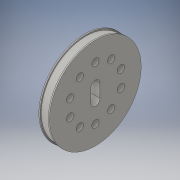
# Autodesk Inventor part: msheehan_wheel_small
Saved by Autodesk Inventor 2016 (Build 200138000, 138)
## iProperties
Created: 2017-09-05
Part Number: msheehan_wheel_small
Material: Generic
Document SubType Name: Modeling
Designer: Student
Density: 1 g/cm^3
Appearance: Default
Author: Student
Autodesk Inventor part; units mm, degrees
sketch "Sketch1" plane through (0, 0, 0) normal (1, 0, 0) x (0, 1, 0)
  circle A0 centre (0, 0) radius 23.368
  dimension "d0" = 46.736
  constraints: 1 centre point, 1 coincident
  measures "d0" diameter of A0
extrude "Extrusion1" add sketch "Sketch1" along normal blind 5.588
ref_plane "Work Plane2" through (5.588, 0, 0) normal (1, 0, 0) x (0, 0, -1)
sketch "Sketch3" plane through (5.588, 0, 0) normal (1, 0, 0) x (0, 0, -1)
  line L0 (0, -3.4925) -> (0, 3.4925) construction
  line L1 (2.413, -3.4925) -> (2.413, 3.4925)
  line L2 (-2.413, 3.4925) -> (-2.413, -3.4925)
  arc A0 (-2.413, -3.4925) -> (2.413, -3.4925) centre (0, -3.4925) ccw
  arc A1 (2.413, 3.4925) -> (-2.413, 3.4925) centre (0, 3.4925) ccw
  point P0 (0, 0)
  dimension "d8" = 3.4925
  dimension "d9" = 4.826
  constraints: 8 end point, 4 point on circle, 4 tangent, 2 centre point, 1 midpoint, 1 parallel, 1 vertical
  measures "d8" distance of point (0, 0) L0.end
  measures "d9" diameter of A1
extrude "Extrusion2" cut sketch "Sketch3" against normal blind 5.08
ref_plane "Work Plane3" through (5.588, 0, 0) normal (1, 0, 0) x (0, 0, -1)
sketch "Sketch6" plane through (5.588, 0, 0) normal (1, 0, 0) x (0, 0, -1)
  line L0 (0, 0) -> (0, 13.97)
  circle A0 centre (0, 13.97) radius 1.905
  circle A1 centre (-8.2114, 11.302) radius 1.905
  circle A2 centre (-13.2863, 4.317) radius 1.905
  circle A3 centre (-13.2863, -4.317) radius 1.905
  circle A4 centre (-8.2114, -11.302) radius 1.905
  circle A5 centre (0, -13.97) radius 1.905
  circle A6 centre (8.2114, -11.302) radius 1.905
  circle A7 centre (13.2863, -4.317) radius 1.905
  circle A8 centre (13.2863, 4.317) radius 1.905
  circle A9 centre (8.2114, 11.302) radius 1.905
  dimension "d16" = 13.97
  dimension "d17" = 3.81
  dimension "d20" = 360
  constraints: 10 centre point, 2 coincident, 2 end point, 1 vertical, 21 other
  measures "d16" distance of L0.start L0.end
  measures "d17" diameter of A0
extrude "Extrusion3" cut sketch "Sketch6" against normal blind 25.4
ref_plane "Work Plane1" through (5.588, 0, 0) normal (1, 0, 0) x (0, 0, -1)
sketch "Sketch7" plane through (5.588, 0, 0) normal (1, 0, 0) x (0, 0, -1)
  line L0 (0, 0) -> (0, -23.749) construction
  circle A0 centre (0, 0) radius 23.749 projected
  dimension "d24" = 23.749
  constraints: 2 end point, 1 vertical, 1 vertical alignment, 1 other
  measures "d24" distance of L0.start L0.end
sketch "Sketch8" plane through (0, 0, 0) normal (0, 1, 0) x (-1, 0, 0)
  line L0 (0, -23.368) -> (0, 23.368) projected
  line L1 (0, -23.368) -> (0, -24.003)
  line L2 (0, -24.003) -> (-0.635, -24.003)
  line L3 (-0.635, -24.003) -> (-0.635, -23.368)
  line L4 (-0.635, -23.368) -> (0, -23.368)
  line L5 (0, -23.368) -> (-5.588, -23.368) projected
  line L6 (-0.635, -23.368) -> (0, -23.368)
  line L7 (-5.588, -23.368) -> (-5.588, -24.003)
  line L8 (-5.588, -24.003) -> (-4.953, -24.003)
  line L9 (-4.953, -24.003) -> (-4.953, -23.368)
  line L10 (-4.953, -23.368) -> (-5.588, -23.368)
  line L11 (0, 0) -> (-5.8379, 0)
  dimension "d25" = 0.635
  dimension "d26" = 0.635
  dimension "d27" = 0.635
  dimension "d28" = 0.635
  constraints: 20 end point, 5 perpendicular, 2 collinear, 2 vertical, 1 horizontal, 1 point on line
  measures "d25" distance of L0.start L1.end
  measures "d26" distance of L1.end L2.end
  measures "d27" distance of L5.end L7.end
  measures "d28" distance of L7.end L8.end
revolve "Revolution2" add sketch "Sketch8" angle 360 about axis through (0, 0, 0) along (1, 0, 0)
body "Solid1"
